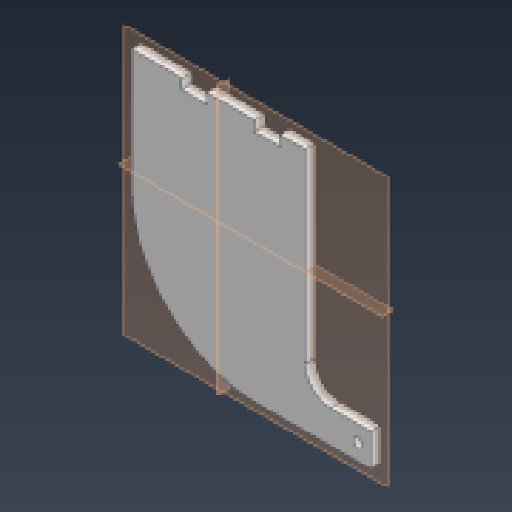
# Autodesk Inventor part: дополнительное_ребро_жёсткости
Saved by Autodesk Inventor 2023.2 (Build 272271030, 271C)
## iProperties
Created: 2026-01-07
Part Number: дополнительное_ребро_жёсткости
Material: Типовые
Document SubType Name: Modeling
Designer: Олег Коноваленко
Density: 1 g/cm^3
Appearance: По умолчанию
Author: Олег Коноваленко
Autodesk Inventor part; units mm, degrees
sketch "Эскиз2" plane through (0, 0, 0) normal (0, 0, 1) x (1, 0, 0)
  line L0 (-34.5, -42) -> (34.5, -42)
  line L1 (34.5, -42) -> (34.5, 42)
  line L2 (34.5, 42) -> (-34.5, 42)
  line L3 (-34.5, 42) -> (-34.5, -42)
  line L4 (-34.5, -42) -> (34.5, 42) construction
  line L5 (34.5, -42) -> (-34.5, 42) construction
  line L6 (-34.5, -42) -> (50.5, -42)
  line L7 (50.5, -42) -> (50.5, -55)
  line L8 (50.5, -55) -> (-34.5, -55)
  line L9 (-34.5, -55) -> (-34.5, -42)
  circle A0 centre (15.5, -5) radius 50
  line L10 (60.5, -42) -> (60.5, -55) projected
  line L11 (50.5, -42) -> (60.5, -42) projected
  line L12 (50.5, -55) -> (50.5, -42) projected
  line L13 (60.5, -55) -> (50.5, -55) projected
  line L14 (50.5, -55) -> (60.5, -42) construction
  line L15 (50.5, -42) -> (60.5, -55) construction
  circle A1 centre (55.5, -48.5) radius 2
  circle A2 centre (55.5, -48.5) radius 2 projected
  point P0 (0, 0)
  point P1 (34.5, -42)
  point P2 (-34.5, -37)
  point P3 (15.5, -55)
  point P4 (-18.1303, -42)
  point P5 (50.5, -42.7071)
  point P6 (-34.5, -5)
  point P7 (-1.5587, 42)
  point P8 (34.5, 41.2493)
  dimension "d7" = 69
  dimension "d8" = 84
  dimension "d9" = 85
  dimension "d10" = 13
  dimension "d15" = 100
  dimension "d27" = 4
  constraints: 24 end point, 4 parallel, 3 midpoint, 2 centre point, 2 horizontal, 2 perpendicular, 2 point on line, 2 tangent
  measures "d7" distance of L1.end L2.end
  measures "d8" distance of L0.end L1.end
  measures "d9" distance of L7.end L8.end
  measures "d10" distance of L8.end L6.start
  measures "d15" diameter of A0
  measures "d27" diameter of A1
extrude "Выдавливание2" add sketch "Эскиз2" along normal mid plane 4 contours A0 L2 L1 L0 | L0 L6 A0 | L3 L2 A0 | A0 L6 L7 L8 | A0 L2 L1 | L7 L11 L10 L13
sketch "Эскиз3" plane through (0, 0, 2) normal (0, 0, 1) x (1, 0, 0)
  line L0 (34.5, 42) -> (-34.5, 42) projected
  line L1 (-14.5, 42) -> (-4.5, 42)
  line L2 (-4.5, 42) -> (-4.5, 38)
  line L3 (-4.5, 38) -> (-14.5, 38)
  line L4 (-14.5, 38) -> (-14.5, 42)
  line L5 (14.5, 42) -> (24.5, 42)
  line L6 (24.5, 42) -> (24.5, 38)
  line L7 (24.5, 38) -> (14.5, 38)
  line L8 (14.5, 38) -> (14.5, 42)
  line L9 (-34.5, 42) -> (-34.5, -5) projected
  line L10 (34.5, -42) -> (34.5, 42) projected
  point P0 (0, 0)
  point P1 (-34.5, -37)
  point P2 (-14.5, 40)
  point P3 (24.5, 42)
  point P4 (-4.5, 42)
  point P5 (-34.5, -69)
  dimension "d16" = 10
  dimension "d17" = 4
  dimension "d18" = 20
  dimension "d19" = 10
  constraints: 16 end point, 4 parallel, 3 point on line, 2 horizontal, 2 perpendicular, 1 collinear, 1 midpoint
  measures "d16" distance of L2.end L3.end
  measures "d17" distance of L3.end L1.start
  measures "d18" distance from line of L9 point (-14.5, 40)
  measures "d19" distance between parallel lines of L10 L6
extrude "Выдавливание3" cut sketch "Эскиз3" against normal up to next
fillet "Сопряжение1" radius 10 1 edges at (34.5, -42, 0)
sketch "Эскиз6" plane through (0, 0, 2) normal (0, 0, 1) x (1, 0, 0)
  line L0 (-25.95, 38) -> (-25.95, 42) projected
  line L1 (-23.05, 42) -> (-23.05, 38) projected
  line L2 (3.55, 38) -> (3.55, 42) projected
  line L3 (6.45, 42) -> (6.45, 38) projected
  line L4 (-25.95, 40) -> (-23.05, 40) construction
  line L5 (3.55, 40) -> (6.45, 40) construction
  circle A0 centre (-24.5, 40) radius 1.5
  circle A1 centre (5, 40) radius 1.5
  point P0 (0, 0)
  point P1 (6.45, 40.3841)
  point P2 (3.55, 40.3841)
  point P3 (3.55, 39.6159)
  point P4 (6.45, 39.6159)
  point P5 (-23.05, 40.3841)
  point P6 (-25.95, 40.3841)
  point P7 (-25.95, 39.6159)
  point P8 (-23.05, 39.6159)
  dimension "d28" = 3
  constraints: 6 midpoint, 4 end point, 2 centre point, 1 equal radius
  measures "d28" diameter of A0
extrude "Выдавливание6" cut sketch "Эскиз6" against normal up to next contours L0 A0 L1 | L2 A1 L3
sketch "Эскиз7" plane through (0, 0, -2) normal (0, 0, -1) x (-1, 0, 0)
  line L0 (0, -15) -> (0, 15) construction
  line L1 (10, -15) -> (10, 15)
  line L2 (-10, 15) -> (-10, -15)
  arc A0 (-10, -15) -> (10, -15) centre (0, -15) ccw
  arc A1 (10, 15) -> (-10, 15) centre (0, 15) ccw
  point P0 (0, 0)
  dimension "d31" = 10
  dimension "d32" = 30
  constraints: 8 end point, 4 point on circle, 4 tangent, 2 centre point, 1 midpoint, 1 parallel, 1 vertical
  measures "d31" distance from line of L1 point (0, 0)
  measures "d32" distance of L0.start L0.end
extrude "Выдавливание7" cut sketch "Эскиз7" against normal up to next
